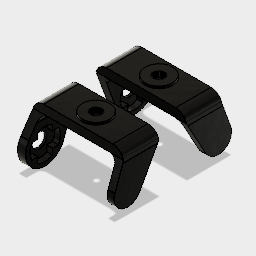
servo_bracket_hip (Autodesk Fusion 360 design; units mm, degrees)
Autodesk Fusion 360 part; units mm, degrees
note: some values were not read from the file. Set by a fixed rule: which sketch regions a step uses.
sketch "スケッチ1" plane through (0, 0, 0) normal (0, 1, 0) x (1, 0, 0)
  line L0 (16.6, -6.5) -> (-16.6, -6.5)
  line L1 (-16.6, -6.5) -> (-16.6, 6.5)
  line L2 (-16.6, 6.5) -> (16.6, 6.5)
  line L3 (16.6, 6.5) -> (16.6, -6.5)
  line L4 (16.6, -6.5) -> (-16.6, 6.5) construction
  line L5 (-16.6, -6.5) -> (16.6, 6.5) construction
  circle A0 centre (0, 0) radius 5.45
  circle A1 centre (0, 0) radius 2.6
  line L6 (0, 0) -> (0, 3.71)
  line L7 (0, 0) -> (-3.71, 0) construction
  line L8 (0, 0) -> (3.71, 0)
  line L9 (0, 0) -> (3.71, 0) construction
  line L10 (0, 3.71) -> (-3.71, 0)
  line L11 (-3.71, 0) -> (0, -3.71)
  line L12 (0, -3.71) -> (3.71, 0)
  line L13 (3.71, 0) -> (0, 3.71)
  line L14 (0, 3.71) -> (-1.5229, 5.2329)
  line L15 (0, 3.71) -> (1.5229, 5.2329)
  line L16 (3.71, 0) -> (5.2329, -1.5229)
  line L17 (3.71, 0) -> (5.2329, 1.5229)
  line L18 (0, -3.71) -> (1.5229, -5.2329)
  line L19 (0, -3.71) -> (-1.5229, -5.2329)
  line L20 (-3.71, 0) -> (-5.2329, -1.5229)
  line L21 (-3.71, 0) -> (-5.2329, 1.5229)
  dimension "d1" = 33.2
  dimension "d2" = 13
  dimension "d3" = 10.9
  dimension "d4" = 5.2
  dimension "d5" = 90
  dimension "d6" = 3.71
  dimension "d7" = 3.71
  measures "d1" distance of L1.end L2.end
  measures "d2" distance of L0.end L1.end
  measures "d3" diameter of A0
  measures "d4" diameter of A1
  measures "d5" angle of L6 L7
  measures "d6" distance of A0.centre L6.end
  measures "d7" distance of A0.centre L8.end
extrude "押し出し1" add sketch "スケッチ1" along normal blind 3.2 contours L0 L1 L2 L3 | A0 L16 L17 | A0 L14 L15 | A0 L18 L19 | A0 L20 L21 makes body 1
extrude "押し出し2" add sketch "スケッチ1" along normal blind 2.1 contours A0 L13 L15 L17 | A0 L12 L16 L18 | A1 L6 L8 L10 L11 L12 | A1 L6 L8 L13 | A0 L10 L14 L21 | A0 L11 L19 L20 bodies 1
ref_plane "作業平面1" through (-16.6, 1.6, 0) normal (-1, 0, 0) x (0, 0, 1)
ref_plane "作業平面2" through (16.6, 1.6, 0) normal (1, 0, 0) x (0, 0, -1)
sketch "スケッチ3" plane through (-16.6, 1.6, 0) normal (-1, 0, 0) x (0, 0, -1)
  line L0 (6.5, -1.6) -> (-5, -1.6)
  line L1 (6.5, -1.6) -> (18.5, -1.6) construction
  line L2 (-5, -1.6) -> (-5, 12.2)
  line L3 (-5, -1.6) -> (-18.3, -1.6) construction
  circle A0 centre (-5, 12.2) radius 2.6
  circle A1 centre (-5, 12.2) radius 7.15
  line L4 (-6.5, 1.6) -> (-10.9381, 8.2174)
  line L5 (6.5, 1.6) -> (1.7133, 14.6604)
  line L6 (-6.5, 1.6) -> (6.5, 1.6)
  point P0 (6.5, -1.6)
  point P1 (-5, 12.2)
  point P2 (-6.5, 1.6)
  point P3 (6.5, 1.6)
  dimension "d20" = 180
  dimension "d21" = 11.5
  dimension "d22" = 90
  dimension "d23" = 13.8
  dimension "d24" = 5.2
  dimension "d28" = 14.3
  measures "d20" angle of L0 L1
  measures "d21" distance of P0 L0.end
  measures "d22" angle of L2 L3
  measures "d23" distance of L0.end P1
  measures "d24" diameter of A0
  measures "d28" diameter of A1
extrude "押し出し3" add sketch "スケッチ3" against normal blind 3 bodies 1
sketch "スケッチ5" plane through (-16.6, 1.6, 0) normal (-1, 0, 0) x (0, 0, -1)
  circle A0 centre (-5, 12.2) radius 5.55
  line L0 (-2.3, 14.9) -> (-7.7, 14.9)
  line L1 (-7.7, 14.9) -> (-7.7, 9.5)
  line L2 (-7.7, 9.5) -> (-2.3, 9.5)
  line L3 (-2.3, 9.5) -> (-2.3, 14.9)
  line L4 (-2.3, 14.9) -> (-7.7, 9.5) construction
  line L5 (-7.7, 14.9) -> (-2.3, 9.5) construction
  line L6 (-7.7, 14.9) -> (-9.849, 14.9)
  line L7 (-7.7, 14.9) -> (-7.7, 17.049)
  line L8 (-7.7, 9.5) -> (-9.849, 9.5)
  line L9 (-7.7, 9.5) -> (-7.7, 7.351)
  line L10 (-2.3, 9.5) -> (-2.3, 7.351)
  line L11 (-2.3, 9.5) -> (-0.151, 9.5)
  line L12 (-2.3, 14.9) -> (-0.151, 14.9)
  line L13 (-2.3, 14.9) -> (-2.3, 17.049)
  point P0 (-5, 12.2)
  point P1 (-5, 12.2)
  dimension "d32" = 11.1
  dimension "d33" = 5.4
  dimension "d34" = 5.4
  measures "d32" diameter of A0
  measures "d33" distance of L1.end L2.end
  measures "d34" distance of L0.end L1.end
extrude "押し出し4" cut sketch "スケッチ5" against normal blind 4.5 contours A0 L3 L11 L12 | A0 L0 L7 L13 | L0 L1 L2 L3 | A0 L2 L9 L10 | A0 L1 L6 L8 bodies 1
extrude "押し出し5" add sketch "スケッチ5" against normal blind 0.9 contours A0 L3 L11 L12 | A0 L0 L7 L13 | L0 L1 L2 L3 | A0 L2 L9 L10 | A0 L1 L6 L8 bodies 1
extrude "押し出し6" cut sketch "スケッチ3" against normal blind 1.5 contours A0 bodies 1
sketch "スケッチ6" plane through (16.6, 1.6, 0) normal (1, 0, 0) x (0, 0, -1)
  circle A0 centre (-5, -12.2) radius 2
  circle A1 centre (-5, -12.2) radius 5
  line L0 (-6.5, -1.6) -> (6.5, -1.6)
  line L1 (6.5, -1.6) -> (6.5, 1.6)
  line L2 (6.5, 1.6) -> (-6.5, 1.6)
  line L3 (-6.5, 1.6) -> (-6.5, -1.6)
  line L4 (-6.5, -1.6) -> (-9.7048, -10.5073)
  line L5 (-0.151, -14.9) -> (-2.3, -14.9)
  line L6 (6.5, -1.6) -> (-0.6138, -14.6002)
  point P0 (-5, -12.2)
  point P1 (-6.5, -1.6)
  point P2 (6.5, 1.6)
  point P3 (6.5, -1.6)
  dimension "d43" = 4
  dimension "d44" = 10
  measures "d43" diameter of A0
  measures "d44" diameter of A1
extrude "押し出し7" add sketch "スケッチ6" against normal blind 2.6 contours A1 | A1 L0 L4 L6 bodies 1
extrude "押し出し8" add sketch "スケッチ6" against normal blind 0.8 contours A0 bodies 1
sketch "スケッチ7" plane through (0, 3.2, 0) normal (0, 1, 0) x (-1, 0, 0)
  arc A0 (5.2329, 1.5229) -> (1.5229, 5.2329) centre (0, 0) ccw
  line L0 (5.2329, 1.5229) -> (3.71, 0)
  line L1 (3.71, 0) -> (5.2329, -1.5229)
  arc A1 (1.5229, -5.2329) -> (5.2329, -1.5229) centre (0, 0) ccw
  line L2 (1.5229, -5.2329) -> (0, -3.71)
  line L3 (0, -3.71) -> (-1.5229, -5.2329)
  arc A2 (-5.2329, -1.5229) -> (-1.5229, -5.2329) centre (0, 0) ccw
  line L4 (-5.2329, -1.5229) -> (-3.71, 0)
  line L5 (-3.71, 0) -> (-5.2329, 1.5229)
  arc A3 (-1.5229, 5.2329) -> (-5.2329, 1.5229) centre (0, 0) ccw
  line L6 (-1.5229, 5.2329) -> (0, 3.71)
  line L7 (0, 3.71) -> (1.5229, 5.2329)
  line L8 (-16.6, -6.5) -> (16.6, -6.5)
  line L9 (16.6, -6.5) -> (16.6, 6.5)
  line L10 (16.6, 6.5) -> (-16.6, 6.5)
  line L11 (-16.6, 6.5) -> (-16.6, -6.5)
  circle A4 centre (0, 0) radius 1.5
  circle A5 centre (0, 0) radius 0.8
  dimension "d49" = 3
  dimension "d50" = 1.6
  measures "d49" diameter of A4
  measures "d50" diameter of A5
extrude "押し出し9" add sketch "スケッチ7" against normal blind 3.2 contours A0 L0 L1 A1 L2 L3 A2 L4 L5 A3 L6 L7 | A4 bodies 1
sketch "スケッチ8" plane through (0, 3.2, 0) normal (0, 1, 0) x (-1, 0, 0)
  circle A0 centre (0, 0) radius 0.8
  line L0 (-16.6, -6.5) -> (16.6, -6.5)
  line L1 (16.6, -6.5) -> (16.6, 6.5)
  line L2 (16.6, 6.5) -> (-16.6, 6.5)
  line L3 (-16.6, 6.5) -> (-16.6, -6.5)
  circle A1 centre (0, 0) radius 1.6 construction
  circle A2 centre (0, 0) radius 2.1 construction
  line L4 (0, 1.6) -> (-0.6508, 1.4617)
  line L5 (-0.6508, 1.4617) -> (-1.189, 1.0706)
  line L6 (-1.189, 1.0706) -> (-1.5217, 0.4944)
  line L7 (-1.5217, 0.4944) -> (-1.5912, -0.1672)
  line L8 (-1.5912, -0.1672) -> (-1.3856, -0.8)
  line L9 (-1.3856, -0.8) -> (-0.9405, -1.2944)
  line L10 (-0.9405, -1.2944) -> (-0.3327, -1.565)
  line L11 (-0.3327, -1.565) -> (0.3327, -1.565)
  line L12 (0.3327, -1.565) -> (0.9405, -1.2944)
  line L13 (0.9405, -1.2944) -> (1.3856, -0.8)
  line L14 (1.3856, -0.8) -> (1.5912, -0.1672)
  line L15 (1.5912, -0.1672) -> (1.5217, 0.4944)
  line L16 (1.5217, 0.4944) -> (1.189, 1.0706)
  line L17 (1.189, 1.0706) -> (0.6508, 1.4617)
  line L18 (0.6508, 1.4617) -> (0, 1.6)
  line L19 (0, -2.1) -> (0.8541, -1.9184)
  line L20 (0.8541, -1.9184) -> (1.5606, -1.4052)
  line L21 (1.5606, -1.4052) -> (1.9972, -0.6489)
  line L22 (1.9972, -0.6489) -> (2.0885, 0.2195)
  line L23 (2.0885, 0.2195) -> (1.8187, 1.05)
  line L24 (1.8187, 1.05) -> (1.2343, 1.6989)
  line L25 (1.2343, 1.6989) -> (0.4366, 2.0541)
  line L26 (0.4366, 2.0541) -> (-0.4366, 2.0541)
  line L27 (-0.4366, 2.0541) -> (-1.2343, 1.6989)
  line L28 (-1.2343, 1.6989) -> (-1.8187, 1.05)
  line L29 (-1.8187, 1.05) -> (-2.0885, 0.2195)
  line L30 (-2.0885, 0.2195) -> (-1.9972, -0.6489)
  line L31 (-1.9972, -0.6489) -> (-1.5606, -1.4052)
  line L32 (-1.5606, -1.4052) -> (-0.8541, -1.9184)
  line L33 (-0.8541, -1.9184) -> (0, -2.1)
  line L34 (0, 1.6) -> (-0.4366, 2.0541)
  line L35 (-0.6508, 1.4617) -> (-0.4366, 2.0541)
  line L36 (0, 1.6) -> (0.4366, 2.0541)
  line L37 (0.4366, 2.0541) -> (0.6508, 1.4617)
  line L38 (0.6508, 1.4617) -> (1.2343, 1.6989)
  line L39 (1.2343, 1.6989) -> (1.189, 1.0706)
  line L40 (1.189, 1.0706) -> (1.8187, 1.05)
  line L41 (1.8187, 1.05) -> (1.5217, 0.4944)
  line L42 (1.5217, 0.4944) -> (2.0885, 0.2195)
  line L43 (2.0885, 0.2195) -> (1.5912, -0.1672)
  line L44 (1.5912, -0.1672) -> (1.9972, -0.6489)
  line L45 (1.9972, -0.6489) -> (1.3856, -0.8)
  line L46 (1.3856, -0.8) -> (1.5606, -1.4052)
  line L47 (1.5606, -1.4052) -> (0.9405, -1.2944)
  line L48 (0.8541, -1.9184) -> (0.9405, -1.2944)
  line L49 (0.8541, -1.9184) -> (0.3327, -1.565)
  line L50 (0.3327, -1.565) -> (0, -2.1)
  line L51 (0, -2.1) -> (-0.3327, -1.565)
  line L52 (-0.3327, -1.565) -> (-0.8541, -1.9184)
  line L53 (-0.8541, -1.9184) -> (-0.9405, -1.2944)
  line L54 (-0.9405, -1.2944) -> (-1.5606, -1.4052)
  line L55 (-1.5606, -1.4052) -> (-1.3856, -0.8)
  line L56 (-1.3856, -0.8) -> (-1.9972, -0.6489)
  line L57 (-1.9972, -0.6489) -> (-1.5912, -0.1672)
  line L58 (-1.5912, -0.1672) -> (-2.0885, 0.2195)
  line L59 (-1.5217, 0.4944) -> (-2.0885, 0.2195)
  line L60 (-1.5217, 0.4944) -> (-1.8187, 1.05)
  line L61 (-1.8187, 1.05) -> (-1.189, 1.0706)
  line L62 (-1.189, 1.0706) -> (-1.2343, 1.6989)
  line L63 (-1.2343, 1.6989) -> (-0.6508, 1.4617)
  dimension "d53" = 3.2
  dimension "d54" = 4.2
  measures "d53" diameter of A1
  measures "d54" diameter of A2
extrude "押し出し10" cut sketch "スケッチ8" against normal blind 2 contours L4 L5 L6 L7 L8 L9 L10 L11 L12 L13 L14 L15 L16 L17 L18 | L18 L36 L37 | L4 L34 L35 | L5 L62 L63 | L17 L38 L39 | L6 L60 L61 | L16 L40 L41 | L7 L58 L59 | L15 L42 L43 | L8 L56 L57 | L14 L44 L45 | L9 L54 L55 | L13 L46 L47 | L10 L52 L53 | L12 L48 L49 | L11 L50 L51 bodies 1
sketch "スケッチ9" plane through (0, 0, 0) normal (0, -1, 0) x (1, 0, 0)
  circle A0 centre (0, 0) radius 0.8
  line L0 (14, -6.5) -> (14, 6.5)
  line L1 (14, 6.5) -> (-13.6, 6.5)
  line L2 (-13.6, 6.5) -> (-13.6, -6.5)
  line L3 (-13.6, -6.5) -> (14, -6.5)
  circle A1 centre (0, 0) radius 1.5
  dimension "d57" = 3
  measures "d57" diameter of A1
extrude "押し出し11" cut sketch "スケッチ9" against normal blind 1 contours A1 bodies 1
fillet "フィレット1" radius 2.5 2 edges at (14, 0, 0) (-13.6, 0, 0) on bodies 1
fillet "フィレット2" radius 4 2 edges at (16.6, 3.2, 0) (-16.6, 3.2, 0) on bodies 1
extrude "押し出し12" add 1 faces at (-0.2763, 1.2, 1.2805) along direction (0, 1, 0) blind 0.8 on bodies 1 bodies 1
sketch "スケッチ10" plane through (0, 3.2, 0) normal (0, 1, 0) x (-1, 0, 0)
  line L0 (-1.5912, -0.1672) -> (-2.0885, 0.2195)
  line L1 (-2.0885, 0.2195) -> (-1.5217, 0.4944)
  line L2 (-1.5217, 0.4944) -> (-1.8187, 1.05)
  line L3 (-1.8187, 1.05) -> (-1.189, 1.0706)
  line L4 (-1.189, 1.0706) -> (-1.2343, 1.6989)
  line L5 (-1.2343, 1.6989) -> (-0.6508, 1.4617)
  line L6 (-0.6508, 1.4617) -> (-0.4366, 2.0541)
  line L7 (-0.4366, 2.0541) -> (0, 1.6)
  line L8 (0, 1.6) -> (0.4366, 2.0541)
  line L9 (0.4366, 2.0541) -> (0.6508, 1.4617)
  line L10 (0.6508, 1.4617) -> (1.2343, 1.6989)
  line L11 (1.2343, 1.6989) -> (1.189, 1.0706)
  line L12 (1.189, 1.0706) -> (1.8187, 1.05)
  line L13 (1.8187, 1.05) -> (1.5217, 0.4944)
  line L14 (1.5217, 0.4944) -> (2.0885, 0.2195)
  line L15 (2.0885, 0.2195) -> (1.5912, -0.1672)
  line L16 (1.5912, -0.1672) -> (1.9972, -0.6489)
  line L17 (1.9972, -0.6489) -> (1.3856, -0.8)
  line L18 (1.3856, -0.8) -> (1.5606, -1.4052)
  line L19 (1.5606, -1.4052) -> (0.9405, -1.2944)
  line L20 (0.9405, -1.2944) -> (0.8541, -1.9184)
  line L21 (0.8541, -1.9184) -> (0.3327, -1.565)
  line L22 (0.3327, -1.565) -> (0, -2.1)
  line L23 (0, -2.1) -> (-0.3327, -1.565)
  line L24 (-0.3327, -1.565) -> (-0.8541, -1.9184)
  line L25 (-0.8541, -1.9184) -> (-0.9405, -1.2944)
  line L26 (-0.9405, -1.2944) -> (-1.5606, -1.4052)
  line L27 (-1.5606, -1.4052) -> (-1.3856, -0.8)
  line L28 (-1.3856, -0.8) -> (-1.9972, -0.6489)
  line L29 (-1.9972, -0.6489) -> (-1.5912, -0.1672)
  line L30 (12.6, -6.5) -> (12.6, 6.5)
  line L31 (12.6, 6.5) -> (-12.6, 6.5)
  line L32 (-12.6, 6.5) -> (-12.6, -6.5)
  line L33 (-12.6, -6.5) -> (12.6, -6.5)
  circle A0 centre (0, 0) radius 5
  dimension "d64" = 10
  measures "d64" diameter of A0
extrude "押し出し13" add sketch "スケッチ10" along normal blind 0.8 contours A0 bodies 1
ref_plane "作業平面3" through (0, 1.6, -11.5) normal (0, 0, -1) x (-1, 0, 0)
mirror "ミラー1" about plane through (0, 1.6, -11.5) normal (0, 0, -1) of bodies 1 makes body 2
